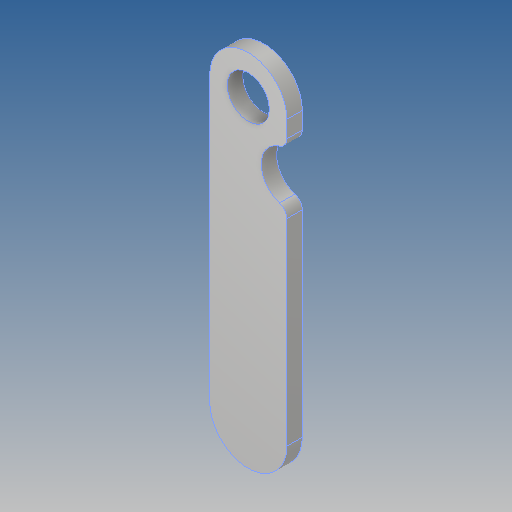
# Autodesk Inventor part: Jambe
Saved by Autodesk Inventor 2018 (Build 220112000, 112)
## iProperties
Created: 2022-03-25
Part Number: Jambe
Material: Aluminum 6061
Document SubType Name: Modeling
Designer: Nathann
Density: 2.7 g/cm^3
Appearance: Aluminum - Flat
Mass: 7.35955 g
Surface Area: 23.7938 cm^2
Volume: 2.72576 cm^3
Author: Nathann
Autodesk Inventor part; units mm, degrees
ref_plane "YZ Plane" through (0, 0, 0) normal (1, 0, 0) x (0, 1, 0)
ref_plane "XZ Plane" through (0, 0, 0) normal (0, 1, 0) x (-1, 0, 0)
ref_plane "XY Plane" through (0, 0, 0) normal (0, 0, 1) x (1, 0, 0)
sketch "Sketch1" plane through (0, 0, 0) normal (0, 0, 1) x (1, 0, 0)
  circle A0 centre (0, 0) radius 4.1
  arc A1 (-7.5, 0) -> (7.5, 0) centre (0, 0) ccw
  circle A2 centre (0, 55) radius 4.1
  arc A3 (7.5, 55) -> (-7.5, 55) centre (0, 55) ccw
  line L0 (-7.5, 55) -> (-7.5, 0)
  circle A4 centre (7.5, 45) radius 5
  line L1 (7.5, 0) -> (7.5, 40)
  line L2 (7.5, 50) -> (7.5, 55)
  dimension "d0" = 55
  dimension "d1" = 15
  dimension "d2" = 8.2
  dimension "d3" = 8.2
  dimension "d4" = 10
  dimension "d5" = 10
  dimension "d8" = 15
  dimension "d10" = 15
  constraints: 6 end point, 6 point on circle, 5 centre point, 3 coincident, 3 tangent, 2 parallel, 2 vertical
  measures "d0" distance of point (0, 0) A2.centre
  measures "d1" diameter of A1
  measures "d2" diameter of A2
  measures "d3" diameter of A0
  measures "d4" diameter of A4
  measures "d5" vertical distance of A2.centre A4.centre
  measures "d8" distance from line of L0 A4.centre
  measures "d10" distance between parallel lines of L0 L1
extrude "Extrusion1" add sketch "Sketch1" along normal blind 3 contours A0 | L0 A3 L2 A4 L1 A1
fillet "Fillet1" radius 2 2 edges at (7.5, 50, 1.5) (7.5, 40, 1.5)
equation "\"d3\" = d2"
equation "\"d5\" = d4"
equation "\"d8\" = d10"
body "Solid1"
